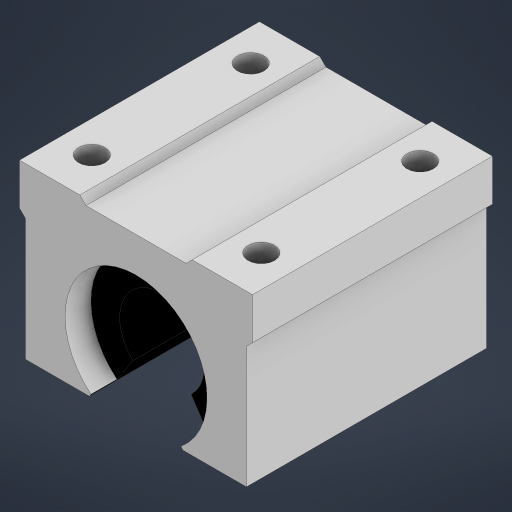
# Autodesk Inventor part: Linear Rail Slider Block
Saved by Autodesk Inventor 2024 (Build 280153000, 153)
## iProperties
Created: 2024-10-26
Part Number: Linear Rail Slider Block
Material: Generic
Document SubType Name: Modeling
Designer: jerem
Density: 1 g/cm^3
Appearance: Default
Author: jerem
Autodesk Inventor part; units mm, degrees
ref_plane "YZ Plane" through (0, 0, 0) normal (1, 0, 0) x (0, 1, 0)
ref_plane "XZ Plane" through (0, 0, 0) normal (0, 1, 0) x (-1, 0, 0)
ref_plane "XY Plane" through (0, 0, 0) normal (0, 0, 1) x (1, 0, 0)
sketch "Sketch1" plane through (0, 0, 0) normal (0, 0, 1) x (1, 0, 0)
  line L0 (-20.85, 0) -> (-20.85, -23)
  line L1 (20.85, -23) -> (20.85, 0)
  line L2 (0, 0) -> (0, -23) construction
  line L3 (-22, 9) -> (-22, 1.15)
  line L4 (-22, 1.15) -> (-20.85, 0)
  line L5 (22, 9) -> (22, 1.15)
  line L6 (22, 1.15) -> (20.85, 0)
  line L7 (0, 0) -> (0, 7.85) construction
  line L8 (-10.6, 9) -> (-9.45, 7.85)
  line L9 (-9.45, 7.85) -> (0, 7.85)
  line L10 (0, 7.85) -> (9.45, 7.85)
  line L11 (9.45, 7.85) -> (10.6, 9)
  line L12 (-22, 9) -> (-10.6, 9)
  line L13 (10.6, 9) -> (22, 9)
  arc A0 (5.5, -18) -> (-5.5, -18) centre (0, -12.1905) ccw
  line L14 (-5.5, -18) -> (5.5, -18) construction
  line L15 (-5.5, -18) -> (-8.8166, -23)
  line L16 (5.5, -18) -> (8.8166, -23)
  line L17 (-20.85, -23) -> (-8.8166, -23)
  line L18 (8.8166, -23) -> (20.85, -23)
  line L19 (8.8166, -23) -> (-8.8166, -23) construction
  arc A1 (8.5116, -22.5401) -> (-8.5116, -22.5401) centre (0, -12.1905) ccw
  point P0 (20.85, -11.5)
  dimension "d1" = 44
  dimension "d3" = 135
  dimension "d4" = 135
  dimension "d5" = 18.9
  dimension "d8" = 23
  dimension "d9" = 135
  dimension "d10" = 23
  dimension "d11" = 1.15
  dimension "d12" = 1.15
  dimension "d13" = 16
  dimension "d14" = 11
  dimension "d16" = 6
  dimension "d17" = 5
  dimension "d18" = 32
  dimension "d19" = 5.4
  constraints: 40 end point, 7 perpendicular, 5 equal length, 5 vertical, 4 point on circle, 4 point on line, 2 centre point, 2 collinear, 2 horizontal, 2 midpoint, 1 coincident
  measures "d1" distance of L3.start L5.start
  measures "d3" angle of L1 L6
  measures "d4" angle of L0 L4
  measures "d5" distance of L10.end L8.end
  measures "d8" distance of L1.start L1.end
  measures "d9" angle of L8 L12
  measures "d10" distance of L2.end L2.start
  measures "d11" distance between parallel lines of L12 L9
  measures "d12" distance between parallel lines of L3 L0
  measures "d13" diameter of A0
  measures "d14" distance of L14.end L14.start
  measures "d16" distance of L14.start L15.end
  measures "d17" distance between parallel lines of L19 L14
  measures "d18" distance between parallel lines of L18 L13
  measures "d19" radial gap between concentric circles of A1 A0
extrude "Extrusion1" add sketch "Sketch1" along normal mid plane 45.3 contours L4 L3 L12 L8 L9 L10 L11 L13 L5 L6 L1 L18 L16 A1 L15 L17 L0
extrude "Extrusion2" add sketch "Sketch1" along normal mid plane 35.5 contours A1 L16 A0 L15
sketch "Sketch2" plane through (-22, 9, 22.65) normal (0, 1, 0) x (1, 0, 0)
  line L0 (0, 45.3) -> (11.4, 45.3) projected
  line L1 (0, 45.3) -> (0, 0) projected
  line L2 (32.6, 45.3) -> (44, 45.3) projected
  line L3 (44, 45.3) -> (44, 0) projected
  circle A0 centre (38, 37.65) radius 2.5
  circle A1 centre (38, 7.65) radius 2.5
  line L4 (38, 37.65) -> (38, 7.65) construction
  line L5 (38, 22.65) -> (44, 22.65) construction
  circle A2 centre (6, 37.65) radius 2.5
  circle A3 centre (6, 7.65) radius 2.5
  line L6 (6, 37.65) -> (6, 7.65) construction
  line L7 (6, 22.65) -> (0, 22.65) construction
  point P0 (22, 22.65)
  dimension "d24" = 5
  dimension "d25" = 5
  dimension "d26" = 30
  dimension "d27" = 5
  dimension "d28" = 5
  dimension "d29" = 30
  dimension "d30" = 32
  constraints: 8 end point, 4 centre point, 4 midpoint, 2 horizontal, 2 vertical, 1 collinear
  measures "d24" diameter of A0
  measures "d25" diameter of A1
  measures "d26" distance of L4.start L4.end
  measures "d27" diameter of A2
  measures "d28" diameter of A3
  measures "d29" distance of L6.start L6.end
  measures "d30" distance between parallel lines of L4 L6
extrude "Extrusion3" cut sketch "Sketch2" against normal blind 15
equation "\"d10\" = d8"
equation "\"d25\" = d24"
equation "\"d28\" = d27"
body "Solid1"
